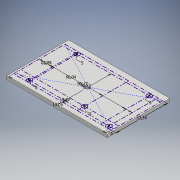
# Autodesk Inventor part: Eletronica - suporteArduino
Saved by Autodesk Inventor 2017 (Build 210142000, 142)
## iProperties
Created: 2020-10-10
Part Number: Eletronica - suporteArduino
Material: Generic
Document SubType Name: Modeling
Designer: ale
Density: 1 g/cm^3
Appearance: Default
Author: ale
Autodesk Inventor part; units mm, degrees
ref_plane "YZ Plane" through (0, 0, 0) normal (1, 0, 0) x (0, 1, 0)
ref_plane "XZ Plane" through (0, 0, 0) normal (0, 1, 0) x (-1, 0, 0)
ref_plane "XY Plane" through (0, 0, 0) normal (0, 0, 1) x (1, 0, 0)
sketch "Sketch1" plane through (0, 0, 0) normal (0, 0, 1) x (1, 0, 0)
  line L0 (-52.5, 32.5) -> (52.5, 32.5)
  line L1 (52.5, 32.5) -> (52.5, -32.5)
  line L2 (52.5, -32.5) -> (-52.5, -32.5)
  line L3 (-52.5, -32.5) -> (-52.5, 32.5)
  line L4 (-52.5, 32.5) -> (52.5, -32.5) construction
  line L5 (52.5, 32.5) -> (-52.5, -32.5) construction
  point P0 (0, 0)
  dimension "d0" = 105
  dimension "d1" = 65
  constraints: 12 end point, 2 midpoint, 2 parallel, 1 horizontal, 1 perpendicular
  measures "d0" distance of L1.end L2.end
  measures "d1" distance of L0.end L1.end
extrude "Extrusion1" add sketch "Sketch1" along normal blind 3
sketch "Sketch2" plane through (0, 0, 3) normal (0, 0, 1) x (1, 0, 0)
  line L0 (-50.8, 26.67) -> (50.8, 26.67)
  line L1 (50.8, 26.67) -> (50.8, -26.67)
  line L2 (50.8, -26.67) -> (-50.8, -26.67)
  line L3 (-50.8, -26.67) -> (-50.8, 26.67)
  line L4 (-50.8, 26.67) -> (50.8, -26.67) construction
  line L5 (50.8, 26.67) -> (-50.8, -26.67) construction
  line L6 (50.8, -24.13) -> (-50.8, -24.13)
  line L7 (-35.56, -26.67) -> (-35.56, 26.67)
  line L8 (50.8, 24.13) -> (-50.8, 24.13)
  circle A0 centre (-35.56, 24.13) radius 2.5
  line L9 (-36.83, -26.67) -> (-36.83, 26.67)
  circle A1 centre (-36.83, -24.13) radius 2.5
  line L10 (45.72, -26.67) -> (45.72, 26.67)
  circle A2 centre (45.72, -24.13) radius 2.5
  line L11 (15.24, -26.67) -> (15.24, 26.67)
  line L12 (50.8, -19.05) -> (-50.8, -19.05)
  circle A3 centre (15.24, -19.05) radius 2.5
  line L13 (39.37, -26.67) -> (39.37, 26.67)
  circle A4 centre (39.37, 24.13) radius 2.5
  point P0 (0, 0)
  dimension "d4" = 101.6
  dimension "d5" = 53.34
  dimension "d6" = 2.54
  dimension "d7" = 15.24
  dimension "d8" = 50.8
  dimension "d9" = 5
  dimension "d10" = 13.97
  dimension "d11" = 5
  dimension "d12" = 96.52
  dimension "d13" = 5
  dimension "d14" = 66.04
  dimension "d15" = 7.62
  dimension "d16" = 5
  dimension "d17" = 90.17
  dimension "d18" = 5
  constraints: 28 end point, 10 parallel, 10 point on line, 5 centre point, 2 midpoint, 1 horizontal, 1 perpendicular
  measures "d4" distance of L1.end L2.end
  measures "d5" distance of L0.end L1.end
  measures "d6" distance between parallel lines of L2 L6
  measures "d7" distance between parallel lines of L3 L7
  measures "d8" distance between parallel lines of L2 L8
  measures "d9" diameter of A0
  measures "d10" distance between parallel lines of L3 L9
  measures "d11" diameter of A1
  measures "d12" distance between parallel lines of L3 L10
  measures "d13" diameter of A2
  measures "d14" distance between parallel lines of L3 L11
  measures "d15" distance between parallel lines of L2 L12
  measures "d16" diameter of A3
  measures "d17" distance between parallel lines of L3 L13
  measures "d18" diameter of A4
body "Solid1"
